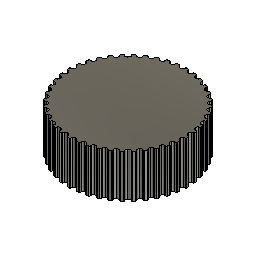
gear_44z (Autodesk Fusion 360 design; units mm, degrees)
Autodesk Fusion 360 part; units mm, degrees
sketch "Sketch1" plane through (0, 0, 0) normal (0, 0, 1) x (1, 0, 0) in component "gt2 pulley"
  circle A0 centre (0, 0) radius 14.0056 construction
  circle A1 centre (0, 0) radius 13.0016 construction
  line L0 (0, 0) -> (0, 14.0056) construction
  line L1 (0, 0) -> (0.9992, 13.97) construction
  line L2 (0, 0) -> (1.4079, 13.9347) construction
  circle A2 centre (0, 0) radius 13.7516 construction
  arc A3 (0.385, 13.6103) -> (0.4492, 13.3227) centre (1.3824, 13.682) ccw
  circle A4 centre (0, 0) radius 13.6016 construction
  arc A5 (0.2379, 13.7496) -> (0, 13.7516) centre (0, 0) ccw
  arc A6 (0.385, 13.6103) -> (0.2379, 13.7496) centre (0.2354, 13.5996) ccw
  arc A7 (0.4492, 13.3227) -> (0.9275, 12.9685) centre (0.9671, 13.5221) ccw
  arc A8 (0, 13.7516) -> (-0.2379, 13.7496) centre (0, 0) ccw
  arc A9 (-0.2379, 13.7496) -> (-0.385, 13.6103) centre (-0.2354, 13.5996) ccw
  arc A10 (-0.4492, 13.3227) -> (-0.385, 13.6103) centre (-1.3824, 13.682) ccw
  arc A11 (-0.9275, 12.9685) -> (-0.4492, 13.3227) centre (-0.9671, 13.5221) ccw
  arc A12 (0.9275, 12.9685) -> (-0.9275, 12.9685) centre (0, 0) ccw
  point P0 (1.3824, 13.682)
  point P1 (0, 13.7516)
  dimension "d18" = 28.0113
  dimension "d19" = 4.091
  dimension "d22" = 1.004
  dimension "d24" = 0.75
  dimension "d26" = 1
  dimension "d27" = 0.15
  dimension "d28" = 0.15
  dimension "d47" = 0.555
  dimension "d52" = 3.812
  constraint coincident A0.centre A1.centre
  constraint coincident A0 L0.end
  constraint vertical L0
  constraint coincident A0 L1.end
  constraint coincident A0 L2.end
  constraint concentric A1 A2
  constraint coincident A1 A7.end
  constraint coincident L1 A7.end
  constraint coincident A2 P0
  constraint coincident L2 P0
  constraint coincident P0 A3.centre
  constraint coincident A2 P1
  constraint coincident L0 P1
  constraint concentric A2 A4
  constraint coincident P1 A5.end
  constraint coincident A4 A6.centre
  constraint coincident A3.start A6.start
  constraint tangent A3 A6
  constraint tangent A3 A7
  constraint symmetric L0 A7.end A11.start
  constraint symmetric L0 A3.start A9.end
  constraint symmetric L0 A3.end A10.start
  constraint symmetric L0 A3 A10
  constraint symmetric L0 A5.start A8.end
  constraint symmetric L0 P1 A5.end
  constraint symmetric L0 A5 A8
  constraint symmetric L0 A6 A9
  constraint symmetric L0 A7 A11
  constraint coincident A1 A11.start
  constraint tangent A1 A7
  constraint coincident L1 A7.centre
  measures "d18" diameter of A0
  measures "d19" angle of L0 L1
  measures "d22" distance of A0 A1
  measures "d24" distance of A1 A2
  measures "d26" radius of A3
  measures "d27" distance of A2 A4
  measures "d28" radius of A6
  measures "d47" radius of A7
extrude "Extrude1" add sketch "Sketch1" along normal blind 10 makes body 1
pattern_circular "C-Pattern1" count 44 over 360 about axis through (0, 0, 1.75) along (0, 0, 1) of bodies 1 makes body 2 at (-2.5618, 12.7468, 6.6667) makes body 3 at (-4.3498, 12.2524, 6.6667) makes body 4 at (-4.7363, 12.1083, 3.3333) makes body 5 at (-7.1158, 10.8816, 6.6667) makes body 6 at (-8.5919, 9.7581, 6.6667) makes body 7 at (-10.2834, 7.9557, 6.6667) makes body 8 at (-11.311, 6.4113, 6.6667) makes body 9 at (-11.5087, 6.0492, 3.3333) makes body 10 at (-12.2524, 4.3498, 3.3333) makes body 11 at (-12.7468, 2.5618, 6.6667) makes body 12 at (-13.0012, -0.1031, 6.6667) makes body 13 at (-12.7468, -2.5618, 6.6667) makes body 14 at (-12.6591, -2.9649, 3.3333) makes body 15 at (-11.7835, -5.4947, 6.6667) makes body 16 at (-11.311, -6.4113, 3.3333) makes body 17 at (-9.3382, -9.0465, 6.6667) makes body 18 at (-7.9557, -10.2834, 6.6667) makes body 19 at (-6.4113, -11.311, 6.6667) makes body 20 at (-6.0492, -11.5087, 3.3333) makes body 21 at (-4.3498, -12.2524, 3.3333) makes body 22 at (-2.5618, -12.7468, 3.3333) makes body 23 at (0.7217, -12.9816, 6.6667) makes body 24 at (2.5618, -12.7468, 6.6667) makes body 25 at (4.3498, -12.2524, 6.6667) makes body 26 at (4.7363, -12.1083, 3.3333) makes body 27 at (7.1158, -10.8816, 6.6667) makes body 28 at (8.5919, -9.7581, 6.6667) makes body 29 at (10.2834, -7.9557, 6.6667) makes body 30 at (11.311, -6.4113, 6.6667) makes body 31 at (11.8692, -5.3071, 6.6667) makes body 32 at (12.2524, -4.3498, 3.3333) makes body 33 at (12.7468, -2.5618, 6.6667) makes body 34 at (13.0012, 0.1031, 6.6667) makes body 35 at (12.7468, 2.5618, 6.6667) makes body 36 at (12.4455, 3.7618, 6.6667) makes body 37 at (11.7835, 5.4947, 6.6667) makes body 38 at (11.311, 6.4113, 3.3333) makes body 39 at (10.2834, 7.9557, 3.3333) makes body 40 at (7.9557, 10.2834, 6.6667) makes body 41 at (6.4113, 11.311, 6.6667) makes body 42 at (6.0492, 11.5087, 3.3333) makes body 43 at (4.3498, 12.2524, 3.3333) makes body 44 at (2.5618, 12.7468, 6.6667)
sketch "Sketch2" plane through (0, 0, 10) normal (0, 0, 1) x (-1, 0, 0)
  arc A0 (-12.5403, -5.3038) -> (-12.6059, -5.4954) centre (-12.4684, -5.4354) ccw
  arc A1 (-12.6059, -5.4954) -> (-12.4082, -5.9282) centre (0, 0) ccw
  arc A2 (-12.4082, -5.9282) -> (-12.2205, -6.0041) centre (-12.2729, -5.8636) ccw
  arc A3 (-11.9322, -5.943) -> (-12.2205, -6.0041) centre (-11.8713, -6.9412) ccw
  arc A4 (-11.4113, -6.231) -> (-11.9322, -5.943) centre (-11.8984, -6.497) ccw
  arc A5 (-12.1819, -4.5436) -> (-11.4113, -6.231) centre (0, 0) ccw
  arc A6 (-12.3053, -5.1259) -> (-12.1819, -4.5436) centre (-12.7019, -4.7376) ccw
  arc A7 (-12.5403, -5.3038) -> (-12.3053, -5.1259) centre (-13.0198, -4.4262) ccw
  circle A8 centre (0, 0) radius 13.0016
  constraint concentric A1 A8
extrude "Extrude2" add sketch "Sketch2" against normal blind 10 contours A5 A8 bodies 1 2 3 4 5 6 7 8 9 10 11 12 13 14 15 16 17 18 19 20 21 22 23 24 25 26 27 28 29 30 31 32 33 34 35 36 37 38 39 40 41 42 43 44
extrude "Extrude4" [suppressed] in component "gt2 pulley"
pattern_circular "C-Pattern7" [suppressed] in component "gt2 pulley"
extrude "Extrude3" [suppressed] in component "gt2 pulley"
pattern_circular "C-Pattern6" [suppressed] in component "gt2 pulley"
extrude "Extrude2'" [suppressed] in component "gt2 pulley"
pattern_circular "C-Pattern5" [suppressed] in component "gt2 pulley"
extrude "Extrude1'" [suppressed] in component "gt2 pulley"
pattern_circular "C-Pattern4" [suppressed] in component "gt2 pulley"
pattern_circular "C-Pattern3" [suppressed] in component "gt2 pulley"
pattern_circular "C-Pattern2" [suppressed] in component "gt2 pulley"
pattern_circular "C-Pattern1'" [suppressed] in component "gt2 pulley"
copy_body "Body->Comp1" [suppressed] in component "Component"
copy_body "Body->Comp2" [suppressed] in component "Component'"
copy_body "Body->Comp3" [suppressed] in component "Component''"
copy_body "Body->Comp4" [suppressed] in component "Component'''"
copy_body "Body->Comp5" [suppressed] in component "Component''''"
copy_body "Body->Comp6" [suppressed] in component "Component'''''"
copy_body "Body->Comp7" [suppressed] in component "Component''''''"
copy_body "Body->Comp8" [suppressed] in component "Component'''''''"
copy_body "Body->Comp9" [suppressed] in component "Component''''''''"
copy_body "Body->Comp10" [suppressed] in component "Component'''''''''"
copy_body "Body->Comp11" [suppressed] in component "Component''''''''''"
copy_body "Body->Comp12" [suppressed] in component "Component'''''''''''"
copy_body "Body->Comp13" [suppressed] in component "Component''''''''''''"
copy_body "Body->Comp14" [suppressed] in component "Component'''''''''''''"
copy_body "Body->Comp15" [suppressed] in component "Component''''''''''''''"
copy_body "Body->Comp16" [suppressed] in component "Component'''''''''''''''"
copy_body "Body->Comp17" [suppressed] in component "Component''''''''''''''''"
copy_body "Body->Comp18" [suppressed] in component "Component'''''''''''''''''"
copy_body "Body->Comp19" [suppressed] in component "Component''''''''''''''''''"
copy_body "Body->Comp20" [suppressed] in component "Component'''''''''''''''''''"
component "gt2 pulley" placed x (1, 0, 0) y (0, 1, 0) z (0, 0, 1) at (0, 0, 0)
equation "NumTeeth = 44" comment "min 20"
equation "ToothPitch = 2 mm"
equation "PullyDia = NumTeeth * ToothPitch / PI"
equation "ToothAng = ( ( 360 / NumTeeth ) * 1 deg )"
equation "TransOffsetAngle = ToothAng * 0.2"
equation "Sholulder_Radius = 0.15 mm"
equation "Root_Radius = 0.555 mm"
equation "TransRadius = 1 mm"
equation "ToolHeight = 0.75 mm"
equation "PLD = 0.254 mm"
equation "d18 = PullyDia"
equation "d19 = ToothAng / 2"
equation "d22 = PLD + ToolHeight"
equation "d24 = ToolHeight"
equation "d26 = TransRadius"
equation "d27 = Sholulder_Radius"
equation "d31 = NumTeeth"
equation "d33 = NumTeeth"
equation "d35 = NumTeeth"
equation "d37 = NumTeeth"
equation "d41 = NumTeeth"
equation "d45 = NumTeeth"
equation "d47 = Root_Radius"
equation "d50 = NumTeeth"
